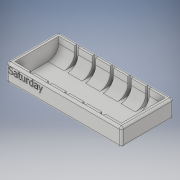
# Autodesk Inventor part: Saturday
Saved by Autodesk Inventor 2019.4 (Build 234330000, 330)
## iProperties
Created: 2020-10-20
Part Number: Saturday
Material: Generic
Document SubType Name: Modeling
Designer: daanswinters
Density: 1 g/cm^3
Appearance: Default
Author: daanswinters
Autodesk Inventor part; units mm, degrees
ref_plane "YZ Plane" through (0, 0, 0) normal (1, 0, 0) x (0, 1, 0)
ref_plane "XZ Plane" through (0, 0, 0) normal (0, 1, 0) x (-1, 0, 0)
ref_plane "XY Plane" through (0, 0, 0) normal (0, 0, 1) x (1, 0, 0)
sketch "Sketch1" plane through (0, 0, 0) normal (0, 0, 1) x (1, 0, 0)
  line L0 (55, -8.5) -> (-55, -8.5)
  line L1 (-55, -8.5) -> (-55, 8.5)
  line L2 (-55, 8.5) -> (55, 8.5)
  line L3 (55, 8.5) -> (55, -8.5)
  line L4 (55, -8.5) -> (-55, 8.5) construction
  line L5 (-55, -8.5) -> (55, 8.5) construction
  point P0 (0, 0)
  dimension "d0" = 110
  dimension "d1" = 17
  constraints: 12 end point, 2 midpoint, 2 parallel, 1 horizontal, 1 perpendicular
  measures "d0" distance of L1.end L2.end
  measures "d1" distance of L0.end L1.end
extrude "Extrusion1" add sketch "Sketch1" along normal blind 50
sketch "Sketch2" plane through (-55, 8.5, 0) normal (0, 1, 0) x (1, 0, 0)
  line L0 (0, 0) -> (0, -50) projected
  line L1 (110, -50) -> (0, -50)
  line L2 (0, -50) -> (0, 0)
  line L3 (0, 0) -> (110, 0)
  line L4 (110, 0) -> (110, -50)
  line L5 (110, -50) -> (0, 0) construction
  line L6 (0, -50) -> (110, 0) construction
  line L7 (106, -46) -> (106, -4)
  line L8 (4, -4) -> (4, -46)
  line L9 (56.15, -2) -> (53.85, -2)
  line L10 (53.85, -48) -> (56.15, -48)
  line L11 (56.15, -2) -> (53.85, -48) construction
  line L12 (53.85, -2) -> (56.15, -48) construction
  line L13 (73.15, -2) -> (70.85, -2)
  line L14 (70.85, -48) -> (73.15, -48)
  line L15 (73.15, -2) -> (70.85, -48) construction
  line L16 (70.85, -2) -> (73.15, -48) construction
  line L17 (0, -25) -> (110, -25) construction
  line L18 (87.85, -2) -> (90.15, -2)
  line L19 (90.15, -48) -> (87.85, -48)
  line L20 (87.85, -2) -> (90.15, -48) construction
  line L21 (90.15, -2) -> (87.85, -48) construction
  line L22 (36.85, -2) -> (39.15, -2)
  line L23 (39.15, -48) -> (36.85, -48)
  line L24 (36.85, -2) -> (39.15, -48) construction
  line L25 (39.15, -2) -> (36.85, -48) construction
  line L26 (19.85, -2) -> (22.15, -2)
  line L27 (22.15, -48) -> (19.85, -48)
  line L28 (19.85, -2) -> (22.15, -48) construction
  line L29 (22.15, -2) -> (19.85, -48) construction
  line L30 (90.15, -2) -> (90.15, -4)
  line L31 (90.15, -46) -> (90.15, -48)
  line L32 (87.85, -48) -> (87.85, -46)
  line L33 (87.85, -4) -> (87.85, -2)
  line L34 (73.15, -48) -> (73.15, -46)
  line L35 (73.15, -4) -> (73.15, -2)
  line L36 (70.85, -2) -> (70.85, -4)
  line L37 (70.85, -46) -> (70.85, -48)
  line L38 (56.15, -4) -> (56.15, -2)
  line L39 (53.85, -2) -> (53.85, -4)
  line L40 (53.85, -46) -> (53.85, -48)
  line L41 (56.15, -48) -> (56.15, -46)
  line L42 (39.15, -2) -> (39.15, -4)
  line L43 (39.15, -46) -> (39.15, -48)
  line L44 (36.85, -48) -> (36.85, -46)
  line L45 (36.85, -4) -> (36.85, -2)
  line L46 (22.15, -2) -> (22.15, -4)
  line L47 (19.85, -48) -> (19.85, -46)
  line L48 (19.85, -4) -> (19.85, -2)
  line L49 (22.15, -46) -> (22.15, -48)
  line L50 (4, -46) -> (19.95, -46)
  line L51 (22.05, -46) -> (36.95, -46)
  line L52 (39.05, -46) -> (53.95, -46)
  line L53 (56.05, -46) -> (70.95, -46)
  line L54 (73.05, -46) -> (87.95, -46)
  line L55 (90.05, -46) -> (106, -46)
  line L56 (106, -4) -> (90.05, -4)
  line L57 (87.95, -4) -> (73.05, -4)
  line L58 (70.95, -4) -> (56.05, -4)
  line L59 (53.95, -4) -> (39.05, -4)
  line L60 (36.95, -4) -> (22.05, -4)
  line L61 (19.95, -4) -> (4, -4)
  point P0 (55, 0)
  point P1 (55, -25)
  point P2 (72, -25)
  point P3 (89, -25)
  point P4 (38, -25)
  point P5 (21, -25)
  dimension "d4" = 65.556
  dimension "d5" = 110
  dimension "d7" = 2.3
  dimension "d8" = 46
  dimension "d9" = 2.3
  dimension "d10" = 46
  dimension "d11" = 0
  dimension "d12" = 2.3
  dimension "d13" = 46
  dimension "d14" = 2.3
  dimension "d15" = 46
  dimension "d16" = 2.3
  dimension "d17" = 46
  dimension "d18" = 17
  dimension "d19" = 17
  dimension "d20" = 17
  dimension "d21" = 17
  dimension "d22" = 2.862
  dimension "d23" = 2.862
  dimension "d24" = 106
  dimension "d25" = 4
  dimension "d26" = 42
  dimension "d27" = 2
  dimension "d28" = 0
  dimension "d29" = 42
  dimension "d30" = 0
  dimension "d31" = 42
  dimension "d32" = 0
  dimension "d33" = 42
  dimension "d34" = 0
  dimension "d35" = 42
  dimension "d36" = 0
  dimension "d37" = 42
  constraints: 122 end point, 73 parallel, 43 point on line, 17 perpendicular, 14 midpoint, 6 horizontal
  measures "d4" angle of L5 L0
  measures "d5" distance between parallel lines of L4 L0
  measures "d7" distance of L10.end L10.start
  measures "d8" distance of L10.start L9.end
  measures "d9" distance of L14.end L14.start
  measures "d10" distance of L14.start L13.end
  measures "d11" distance from line of L17 point (72, -25)
  measures "d12" distance of L19.start L19.end
  measures "d13" distance of L18.end L19.start
  measures "d14" distance of L23.start L23.end
  measures "d15" distance of L22.end L23.start
  measures "d16" distance of L27.start L27.end
  measures "d17" distance of L26.end L27.start
  measures "d18" distance of point (72, -25) point (55, -25)
  measures "d19" distance of point (89, -25) point (72, -25)
  measures "d20" distance of point (38, -25) point (55, -25)
  measures "d21" distance of point (21, -25) point (38, -25)
  measures "d22" angle of L0 L20
  measures "d23" angle of L0 L21
  measures "d24" distance between parallel lines of L7 L0
  measures "d25" distance between parallel lines of L8 L0
  measures "d26" distance between parallel lines of L56 L55
  measures "d27" distance between parallel lines of L56 L18
  measures "d28" distance between parallel lines of L56 L57
  measures "d29" distance between parallel lines of L56 L54
  measures "d30" distance between parallel lines of L56 L58
  measures "d31" distance between parallel lines of L56 L53
  measures "d32" distance between parallel lines of L56 L59
  measures "d33" distance between parallel lines of L56 L52
  measures "d34" distance between parallel lines of L56 L60
  measures "d35" distance between parallel lines of L56 L51
  measures "d36" distance between parallel lines of L56 L61
  measures "d37" distance between parallel lines of L56 L50
extrude "Extrusion2" cut sketch "Sketch2" against normal blind 16 contours L55 L31 L19 L32 L54 L34 L14 L37 L53 L41 L10 L40 L52 L43 L23 L44 L51 L49 L27 L47 L50 L8 L61 L48 L26 L46 L60 L45 L22 L42 L59 L39 L9 L38 L58 L36 L13 L35 L57 L33 L18 L30 L56 L7
fillet "Fillet1" radius 2 12 edges at (-55, 0, 50) (-55, 0, 0) (55, 0, 50) (55, 0, 0) (0, 8.5, 50) (-55, 8.5, 25) (0, 8.5, 0) (55, 8.5, 25) (55, -8.5, 25) (0, -8.5, 50) (-55, -8.5, 25) (0, -8.5, 0)
fillet "Fillet2" radius 10 6 edges at (-43.075, -7.5, 4) (-25.5, -7.5, 4) (-8.5, -7.5, 4) (8.5, -7.5, 4) (25.5, -7.5, 4) (43.075, -7.5, 4)
sketch "Sketch3" plane through (35.15, 8.5, 4) normal (0, 1, 0) x (1, 0, 0)
  line L0 (-70.3, -44) -> (-70.3, -42) projected
  line L1 (-51, 2) -> (-53.3, 2)
  line L2 (-34, 2) -> (-34, 0) projected
  line L3 (-36.3, -44) -> (-36.3, -42) projected
  line L4 (-19.3, -44) -> (-19.3, -42) projected
  line L5 (-2.3, -44) -> (-2.3, -42) projected
  line L6 (0, 2) -> (0, 0) projected
  line L7 (-19.8, 2) -> (-16.5, 2)
  line L8 (-16.5, 2) -> (-16.5, -44)
  line L9 (-16.5, -44) -> (-19.8, -44)
  line L10 (-19.8, -44) -> (-19.8, 2)
  line L11 (-19.8, 2) -> (-16.5, -44) construction
  line L12 (-16.5, 2) -> (-19.8, -44) construction
  line L13 (-2.8, -44) -> (0.5, -44)
  line L14 (0.5, -44) -> (0.5, 2)
  line L15 (0.5, 2) -> (-2.8, 2)
  line L16 (-2.8, 2) -> (-2.8, -44)
  line L17 (-2.8, -44) -> (0.5, 2) construction
  line L18 (0.5, -44) -> (-2.8, 2) construction
  line L19 (-36.8, -44) -> (-33.5, -44)
  line L20 (-33.5, -44) -> (-33.5, 2)
  line L21 (-33.5, 2) -> (-36.8, 2)
  line L22 (-36.8, 2) -> (-36.8, -44)
  line L23 (-36.8, -44) -> (-33.5, 2) construction
  line L24 (-33.5, -44) -> (-36.8, 2) construction
  line L25 (-51, 2) -> (-36.3, 2) projected
  line L26 (-53.8, -44) -> (-50.5, -44)
  line L27 (-50.5, -44) -> (-50.5, 2)
  line L28 (-50.5, 2) -> (-53.8, 2)
  line L29 (-53.8, 2) -> (-53.8, -44)
  line L30 (-53.8, -44) -> (-50.5, 2) construction
  line L31 (-50.5, -44) -> (-53.8, 2) construction
  line L32 (-53.3, -44) -> (-68, -44) projected
  line L33 (-70.8, 2) -> (-67.5, 2)
  line L34 (-67.5, 2) -> (-67.5, -44)
  line L35 (-67.5, -44) -> (-70.8, -44)
  line L36 (-70.8, -44) -> (-70.8, 2)
  line L37 (-70.8, 2) -> (-67.5, -44) construction
  line L38 (-67.5, 2) -> (-70.8, -44) construction
  point P0 (-35.15, 4)
  point P1 (-68, 2)
  point P2 (-17, 2)
  point P3 (-18.15, -21)
  point P4 (-1.15, -21)
  point P5 (-35.15, -21)
  point P6 (-52.15, -21)
  point P7 (-69.15, -21)
  dimension "d42" = 3.3
  dimension "d43" = 46
  dimension "d44" = 3.3
  dimension "d45" = 3.3
  dimension "d46" = 3.3
  dimension "d47" = 3.3
  dimension "d48" = 90
  dimension "d49" = 0.5
  dimension "d50" = 16.5
  dimension "d51" = 33.5
  dimension "d52" = 50.5
  dimension "d53" = 67.5
  dimension "d54" = 46
  dimension "d55" = 0
  dimension "d56" = 53.3
  constraints: 62 end point, 14 parallel, 10 midpoint, 5 horizontal, 5 perpendicular, 3 point on line
  measures "d42" distance of L8.end L9.end
  measures "d43" distance of L7.end L8.end
  measures "d44" distance of L15.end L14.end
  measures "d45" distance of L21.end L20.end
  measures "d46" distance of L28.end L27.end
  measures "d47" distance of L34.end L35.end
  measures "d48" angle of L6 L1
  measures "d49" distance between parallel lines of L6 L14
  measures "d50" distance between parallel lines of L6 L8
  measures "d51" distance between parallel lines of L6 L20
  measures "d52" distance between parallel lines of L6 L27
  measures "d53" distance between parallel lines of L6 L34
  measures "d54" distance between parallel lines of L25 L9
  measures "d55" distance between parallel lines of L15 L25
  measures "d56" distance from line of L1.end L6
extrude "Extrusion3" cut sketch "Sketch3" against normal blind 16
sketch "Sketch4" plane through (0, 0, 50) normal (0, 0, 1) x (1, 0, 0)
  line L0 (-52.9749, 6.5012) -> (53.0345, 6.5012) construction
  line L1 (53.0345, 6.5012) -> (53.0345, -6.5247) construction
  line L2 (53.0345, -6.5247) -> (-52.9749, -6.5247) construction
  line L3 (-52.9749, -6.5247) -> (-52.9749, 6.5012) construction
  spline S0 degree 2 poles (-50.6565, 0.0206) (-51.3189, 0.0206) (-52.2483, 0.2974) (-52.6586, 0.4952) knots 0 0 0 1 2 2 2
  line L4 (-52.6586, 0.4952) -> (-52.6586, 1.5135)
  line L5 (-52.6586, 1.5135) -> (-52.5992, 1.5135)
  spline S1 degree 2 poles (-52.5992, 1.5135) (-52.1988, 1.1378) (-51.1855, 0.7226) (-50.7159, 0.7226) knots 0 0 0 1 2 2 2
  spline S2 degree 2 poles (-50.7159, 0.7226) (-50.0436, 0.7226) (-49.3565, 1.2812) (-49.3565, 1.7409) knots 0 0 0 1 2 2 2
  spline S3 degree 2 poles (-49.3565, 1.7409) (-49.3565, 2.1067) (-49.7173, 2.5615) (-50.1078, 2.6752) knots 0 0 0 1 2 2 2
  spline S4 degree 2 poles (-50.1078, 2.6752) (-50.3896, 2.7542) (-50.8592, 2.863) (-51.2102, 2.952) knots 0 0 0 1 2 2 2
  spline S5 degree 2 poles (-51.2102, 2.952) (-51.5265, 3.036) (-52.0258, 3.2881) (-52.2186, 3.4908) knots 0 0 0 1 2 2 2
  spline S6 degree 2 poles (-52.2186, 3.4908) (-52.4065, 3.6935) (-52.6141, 4.2372) (-52.6141, 4.5931) knots 0 0 0 1 2 2 2
  spline S7 degree 2 poles (-52.6141, 4.5931) (-52.6141, 5.3346) (-51.4573, 6.3381) (-50.5626, 6.3381) knots 0 0 0 1 2 2 2
  spline S8 degree 2 poles (-50.5626, 6.3381) (-50.0485, 6.3381) (-49.1389, 6.1354) (-48.7484, 5.9427) knots 0 0 0 1 2 2 2
  line L6 (-48.7484, 5.9427) -> (-48.7484, 4.9738)
  line L7 (-48.7484, 4.9738) -> (-48.8077, 4.9738)
  spline S9 degree 2 poles (-48.8077, 4.9738) (-49.0994, 5.2407) (-50.009, 5.6362) (-50.5082, 5.6362) knots 0 0 0 1 2 2 2
  spline S10 degree 2 poles (-50.5082, 5.6362) (-51.0718, 5.6362) (-51.7688, 5.1072) (-51.7688, 4.6772) knots 0 0 0 1 2 2 2
  spline S11 degree 2 poles (-51.7688, 4.6772) (-51.7688, 4.2916) (-51.3585, 3.8319) (-50.9729, 3.7281) knots 0 0 0 1 2 2 2
  spline S12 degree 2 poles (-50.9729, 3.7281) (-50.7159, 3.6589) (-49.9694, 3.4809) (-49.7223, 3.4068) knots 0 0 0 1 2 2 2
  spline S13 degree 2 poles (-49.7223, 3.4068) (-49.0945, 3.214) (-48.5112, 2.4379) (-48.5112, 1.8694) knots 0 0 0 1 2 2 2
  spline S14 degree 2 poles (-48.5112, 1.8694) (-48.5112, 1.5085) (-48.8028, 0.8165) (-49.0648, 0.5743) knots 0 0 0 1 2 2 2
  spline S15 degree 2 poles (-49.0648, 0.5743) (-49.3565, 0.3073) (-50.0979, 0.0206) (-50.6565, 0.0206) knots 0 0 0 1 2 2 2
  spline S16 degree 2 poles (-45.1942, 0.6138) (-45.2881, 0.5446) (-45.6045, 0.2974) (-45.7528, 0.2233) knots 0 0 0 1 2 2 2
  spline S17 degree 2 poles (-45.7528, 0.2233) (-45.9555, 0.1145) (-46.3361, 0.0008) (-46.6821, 0.0008) knots 0 0 0 1 2 2 2
  spline S18 degree 2 poles (-46.6821, 0.0008) (-46.9639, 0.0008) (-47.4731, 0.2134) (-47.6659, 0.4062) knots 0 0 0 1 2 2 2
  spline S19 degree 2 poles (-47.6659, 0.4062) (-47.8488, 0.594) (-48.0712, 1.1477) (-48.0712, 1.4542) knots 0 0 0 1 2 2 2
  spline S20 degree 2 poles (-48.0712, 1.4542) (-48.0712, 1.9287) (-47.6708, 2.601) (-47.2358, 2.7938) knots 0 0 0 1 2 2 2
  spline S21 degree 2 poles (-47.2358, 2.7938) (-46.8502, 2.9718) (-45.8022, 3.1052) (-45.1942, 3.1398) knots 0 0 0 1 2 2 2
  line L8 (-45.1942, 3.1398) -> (-45.1942, 3.2881)
  spline S22 degree 2 poles (-45.1942, 3.2881) (-45.1942, 3.5551) (-45.3573, 3.8863) (-45.5056, 3.9802) knots 0 0 0 1 2 2 2
  spline S23 degree 2 poles (-45.5056, 3.9802) (-45.6539, 4.0741) (-46.0791, 4.1334) (-46.3065, 4.1334) knots 0 0 0 1 2 2 2
  spline S24 degree 2 poles (-46.3065, 4.1334) (-46.5734, 4.1334) (-47.2951, 3.9752) (-47.656, 3.822) knots 0 0 0 1 2 2 2
  line L9 (-47.656, 3.822) -> (-47.7005, 3.822)
  line L10 (-47.7005, 3.822) -> (-47.7005, 4.608)
  spline S25 degree 2 poles (-47.7005, 4.608) (-47.4879, 4.6673) (-46.692, 4.8156) (-46.3015, 4.8156) knots 0 0 0 1 2 2 2
  spline S26 degree 2 poles (-46.3015, 4.8156) (-45.827, 4.8156) (-45.1794, 4.6673) (-44.9223, 4.4745) knots 0 0 0 1 2 2 2
  spline S27 degree 2 poles (-44.9223, 4.4745) (-44.6702, 4.2867) (-44.4231, 3.6885) (-44.4231, 3.2585) knots 0 0 0 1 2 2 2
  line L11 (-44.4231, 3.2585) -> (-44.4231, 0.1294)
  line L12 (-44.4231, 0.1294) -> (-45.1942, 0.1294)
  line L13 (-45.1942, 0.1294) -> (-45.1942, 0.6138)
  line L14 (-45.1942, 1.2564) -> (-45.1942, 2.5269)
  spline S28 degree 2 poles (-45.1942, 2.5269) (-45.471, 2.5021) (-46.3065, 2.4181) (-46.5684, 2.339) knots 0 0 0 1 2 2 2
  spline S29 degree 2 poles (-46.5684, 2.339) (-46.8749, 2.2451) (-47.2753, 1.8546) (-47.2753, 1.5085) knots 0 0 0 1 2 2 2
  spline S30 degree 2 poles (-47.2753, 1.5085) (-47.2753, 1.1131) (-46.8304, 0.7127) (-46.4053, 0.7127) knots 0 0 0 1 2 2 2
  spline S31 degree 2 poles (-46.4053, 0.7127) (-46.0445, 0.7127) (-45.4513, 1.0241) (-45.1942, 1.2564) knots 0 0 0 1 2 2 2
  spline S32 degree 2 poles (-41.9564, 0.0404) (-42.5842, 0.0404) (-43.2911, 0.7572) (-43.2911, 1.5333) knots 0 0 0 1 2 2 2
  line L15 (-43.2911, 1.5333) -> (-43.2911, 4.0692)
  line L16 (-43.2911, 4.0692) -> (-43.8101, 4.0692)
  line L17 (-43.8101, 4.0692) -> (-43.8101, 4.7068)
  line L18 (-43.8101, 4.7068) -> (-43.2911, 4.7068)
  line L19 (-43.2911, 4.7068) -> (-43.2911, 6.0218)
  line L20 (-43.2911, 6.0218) -> (-42.5199, 6.0218)
  line L21 (-42.5199, 6.0218) -> (-42.5199, 4.7068)
  line L22 (-42.5199, 4.7068) -> (-41.1012, 4.7068)
  line L23 (-41.1012, 4.7068) -> (-41.1012, 4.0692)
  line L24 (-41.1012, 4.0692) -> (-42.5199, 4.0692)
  line L25 (-42.5199, 4.0692) -> (-42.5199, 1.8892)
  spline S33 degree 2 poles (-42.5199, 1.8892) (-42.5199, 1.5431) (-42.4952, 1.1625) (-42.4112, 0.9994) knots 0 0 0 1 2 2 2
  spline S34 degree 2 poles (-42.4112, 0.9994) (-42.3419, 0.856) (-42.0305, 0.7127) (-41.7636, 0.7127) knots 0 0 0 1 2 2 2
  spline S35 degree 2 poles (-41.7636, 0.7127) (-41.5757, 0.7127) (-41.2248, 0.8264) (-41.1457, 0.861) knots 0 0 0 1 2 2 2
  line L26 (-41.1457, 0.861) -> (-41.1012, 0.861)
  line L27 (-41.1012, 0.861) -> (-41.1012, 0.1689)
  spline S36 degree 2 poles (-41.1012, 0.1689) (-41.3187, 0.1096) (-41.7636, 0.0404) (-41.9564, 0.0404) knots 0 0 0 1 2 2 2
  line L28 (-36.9735, 0.1294) -> (-37.7447, 0.1294)
  line L29 (-37.7447, 0.1294) -> (-37.7447, 0.6336)
  spline S37 degree 2 poles (-37.7447, 0.6336) (-38.1006, 0.3222) (-38.7383, 0.0008) (-39.1338, 0.0008) knots 0 0 0 1 2 2 2
  spline S38 degree 2 poles (-39.1338, 0.0008) (-39.4304, 0.0008) (-39.9593, 0.1986) (-40.1521, 0.4111) knots 0 0 0 1 2 2 2
  spline S39 degree 2 poles (-40.1521, 0.4111) (-40.3498, 0.6237) (-40.5673, 1.2713) (-40.5673, 1.7359) knots 0 0 0 1 2 2 2
  line L30 (-40.5673, 1.7359) -> (-40.5673, 4.7068)
  line L31 (-40.5673, 4.7068) -> (-39.7962, 4.7068)
  line L32 (-39.7962, 4.7068) -> (-39.7962, 2.0968)
  spline S40 degree 2 poles (-39.7962, 2.0968) (-39.7962, 1.731) (-39.7418, 1.2515) (-39.6479, 1.0735) knots 0 0 0 1 2 2 2
  spline S41 degree 2 poles (-39.6479, 1.0735) (-39.5539, 0.8956) (-39.2326, 0.7324) (-38.9311, 0.7324) knots 0 0 0 1 2 2 2
  spline S42 degree 2 poles (-38.9311, 0.7324) (-38.6493, 0.7324) (-38.0116, 1.0538) (-37.7447, 1.2861) knots 0 0 0 1 2 2 2
  line L33 (-37.7447, 1.2861) -> (-37.7447, 4.7068)
  line L34 (-37.7447, 4.7068) -> (-36.9735, 4.7068)
  line L35 (-36.9735, 4.7068) -> (-36.9735, 0.1294)
  line L36 (-33.4292, 3.8813) -> (-33.4688, 3.8813)
  spline S43 degree 2 poles (-33.4688, 3.8813) (-33.5577, 3.906) (-33.7505, 3.9159) (-33.884, 3.9159) knots 0 0 0 1 2 2 2
  spline S44 degree 2 poles (-33.884, 3.9159) (-34.1954, 3.9159) (-34.8084, 3.644) (-35.0852, 3.3771) knots 0 0 0 1 2 2 2
  line L37 (-35.0852, 3.3771) -> (-35.0852, 0.1294)
  line L38 (-35.0852, 0.1294) -> (-35.8564, 0.1294)
  line L39 (-35.8564, 0.1294) -> (-35.8564, 4.7068)
  line L40 (-35.8564, 4.7068) -> (-35.0852, 4.7068)
  line L41 (-35.0852, 4.7068) -> (-35.0852, 4.0247)
  spline S45 degree 2 poles (-35.0852, 4.0247) (-34.665, 4.4004) (-34.0372, 4.7068) (-33.7406, 4.7068) knots 0 0 0 1 2 2 2
  spline S46 degree 2 poles (-33.7406, 4.7068) (-33.622, 4.7068) (-33.5034, 4.697) (-33.4292, 4.6821) knots 0 0 0 1 2 2 2
  line L42 (-33.4292, 4.6821) -> (-33.4292, 3.8813)
  line L43 (-29.3115, 0.1294) -> (-30.0826, 0.1294)
  line L44 (-30.0826, 0.1294) -> (-30.0826, 0.594)
  spline S47 degree 2 poles (-30.0826, 0.594) (-30.2606, 0.4457) (-30.5226, 0.248) (-30.7005, 0.164) knots 0 0 0 1 2 2 2
  spline S48 degree 2 poles (-30.7005, 0.164) (-30.8637, 0.0849) (-31.2146, 0.0008) (-31.447, 0.0008) knots 0 0 0 1 2 2 2
  spline S49 degree 2 poles (-31.447, 0.0008) (-31.8227, 0.0008) (-32.4554, 0.3123) (-32.6778, 0.6138) knots 0 0 0 1 2 2 2
  spline S50 degree 2 poles (-32.6778, 0.6138) (-32.9003, 0.9153) (-33.1475, 1.8051) (-33.1475, 2.3835) knots 0 0 0 1 2 2 2
  spline S51 degree 2 poles (-33.1475, 2.3835) (-33.1475, 2.9866) (-32.836, 3.8665) (-32.5641, 4.1977) knots 0 0 0 1 2 2 2
  spline S52 degree 2 poles (-32.5641, 4.1977) (-32.312, 4.4943) (-31.6052, 4.8354) (-31.2146, 4.8354) knots 0 0 0 1 2 2 2
  spline S53 degree 2 poles (-31.2146, 4.8354) (-30.8735, 4.8354) (-30.3644, 4.6821) (-30.0826, 4.5239) knots 0 0 0 1 2 2 2
  line L45 (-30.0826, 4.5239) -> (-30.0826, 6.5012)
  line L46 (-30.0826, 6.5012) -> (-29.3115, 6.5012)
  line L47 (-29.3115, 6.5012) -> (-29.3115, 0.1294)
  line L48 (-30.0826, 1.2416) -> (-30.0826, 3.8863)
  spline S54 degree 2 poles (-30.0826, 3.8863) (-30.3693, 4.0247) (-30.8241, 4.1285) (-31.0861, 4.1285) knots 0 0 0 1 2 2 2
  spline S55 degree 2 poles (-31.0861, 4.1285) (-31.6793, 4.1285) (-32.3516, 3.2387) (-32.3516, 2.3983) knots 0 0 0 1 2 2 2
  spline S56 degree 2 poles (-32.3516, 2.3983) (-32.3516, 1.5876) (-31.8375, 0.7324) (-31.269, 0.7324) knots 0 0 0 1 2 2 2
  spline S57 degree 2 poles (-31.269, 0.7324) (-30.9675, 0.7324) (-30.3545, 1.0093) (-30.0826, 1.2416) knots 0 0 0 1 2 2 2
  spline S58 degree 2 poles (-25.6436, 0.6138) (-25.7375, 0.5446) (-26.0539, 0.2974) (-26.2022, 0.2233) knots 0 0 0 1 2 2 2
  spline S59 degree 2 poles (-26.2022, 0.2233) (-26.4048, 0.1145) (-26.7855, 0.0008) (-27.1315, 0.0008) knots 0 0 0 1 2 2 2
  spline S60 degree 2 poles (-27.1315, 0.0008) (-27.4133, 0.0008) (-27.9224, 0.2134) (-28.1152, 0.4062) knots 0 0 0 1 2 2 2
  spline S61 degree 2 poles (-28.1152, 0.4062) (-28.2981, 0.594) (-28.5206, 1.1477) (-28.5206, 1.4542) knots 0 0 0 1 2 2 2
  spline S62 degree 2 poles (-28.5206, 1.4542) (-28.5206, 1.9287) (-28.1201, 2.601) (-27.6851, 2.7938) knots 0 0 0 1 2 2 2
  spline S63 degree 2 poles (-27.6851, 2.7938) (-27.2996, 2.9718) (-26.2516, 3.1052) (-25.6436, 3.1398) knots 0 0 0 1 2 2 2
  line L49 (-25.6436, 3.1398) -> (-25.6436, 3.2881)
  spline S64 degree 2 poles (-25.6436, 3.2881) (-25.6436, 3.5551) (-25.8067, 3.8863) (-25.955, 3.9802) knots 0 0 0 1 2 2 2
  spline S65 degree 2 poles (-25.955, 3.9802) (-26.1033, 4.0741) (-26.5284, 4.1334) (-26.7558, 4.1334) knots 0 0 0 1 2 2 2
  spline S66 degree 2 poles (-26.7558, 4.1334) (-27.0227, 4.1334) (-27.7445, 3.9752) (-28.1053, 3.822) knots 0 0 0 1 2 2 2
  line L50 (-28.1053, 3.822) -> (-28.1498, 3.822)
  line L51 (-28.1498, 3.822) -> (-28.1498, 4.608)
  spline S67 degree 2 poles (-28.1498, 4.608) (-27.9372, 4.6673) (-27.1414, 4.8156) (-26.7509, 4.8156) knots 0 0 0 1 2 2 2
  spline S68 degree 2 poles (-26.7509, 4.8156) (-26.2763, 4.8156) (-25.6287, 4.6673) (-25.3717, 4.4745) knots 0 0 0 1 2 2 2
  spline S69 degree 2 poles (-25.3717, 4.4745) (-25.1196, 4.2867) (-24.8724, 3.6885) (-24.8724, 3.2585) knots 0 0 0 1 2 2 2
  line L52 (-24.8724, 3.2585) -> (-24.8724, 0.1294)
  line L53 (-24.8724, 0.1294) -> (-25.6436, 0.1294)
  line L54 (-25.6436, 0.1294) -> (-25.6436, 0.6138)
  line L55 (-25.6436, 1.2564) -> (-25.6436, 2.5269)
  spline S70 degree 2 poles (-25.6436, 2.5269) (-25.9204, 2.5021) (-26.7558, 2.4181) (-27.0178, 2.339) knots 0 0 0 1 2 2 2
  spline S71 degree 2 poles (-27.0178, 2.339) (-27.3243, 2.2451) (-27.7247, 1.8546) (-27.7247, 1.5085) knots 0 0 0 1 2 2 2
  spline S72 degree 2 poles (-27.7247, 1.5085) (-27.7247, 1.1131) (-27.2798, 0.7127) (-26.8547, 0.7127) knots 0 0 0 1 2 2 2
  spline S73 degree 2 poles (-26.8547, 0.7127) (-26.4938, 0.7127) (-25.9006, 1.0241) (-25.6436, 1.2564) knots 0 0 0 1 2 2 2
  line L56 (-20.1961, 4.7068) -> (-22.6578, -1.5563)
  line L57 (-22.6578, -1.5563) -> (-23.4834, -1.5563)
  line L58 (-23.4834, -1.5563) -> (-22.6628, 0.3518)
  line L59 (-22.6628, 0.3518) -> (-24.3237, 4.7068)
  line L60 (-24.3237, 4.7068) -> (-23.4932, 4.7068)
  line L61 (-23.4932, 4.7068) -> (-22.2426, 1.3158)
  line L62 (-22.2426, 1.3158) -> (-20.9969, 4.7068)
  line L63 (-20.9969, 4.7068) -> (-20.1961, 4.7068)
  point P0 (0, 0)
  constraints: 2 other
extrude "Extrusion4" cut sketch "Sketch4" against normal blind 0.5
fillet "Fillet3" radius 10 6 edges at (-43.325, -7.5, 46) (-25.5, -7.5, 46) (-8.5, -7.5, 46) (8.5, -7.5, 46) (25.5, -7.5, 46) (43.325, -7.5, 46)
body "Solid1"
